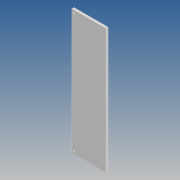
# Autodesk Inventor part: KB33-046-004-005 - Лицевая наклонная пластина
Saved by Autodesk Inventor 2020 (Build 240168000, 168)
## iProperties
Created: 2021-06-25
Part Number: KB33-046-004-005 - Лицевая наклонная пластина
Material: Типовые
Document SubType Name: Modeling
Designer: Петров Иван
Mass: 52.5036 g
Surface Area: 285.592 cm^2
Volume: 52.5036 cm^3
Density: 1 g/cm^3
Appearance: По умолчанию
Author: Петров Иван
Autodesk Inventor part; units mm, degrees
ref_plane "YZ Plane" through (0, 0, 0) normal (1, 0, 0) x (0, 1, 0)
ref_plane "XZ Plane" through (0, 0, 0) normal (0, 1, 0) x (-1, 0, 0)
ref_plane "XY Plane" through (0, 0, 0) normal (0, 0, 1) x (1, 0, 0)
sketch "Эскиз1" plane through (0, 0, 0) normal (0, 0, 1) x (1, 0, 0)
  circle A0 centre (3.6373, -187.3954) radius 1.5 projected
  circle A1 centre (3.6373, 22.3954) radius 1.5 projected
  line L0 (0, 27) -> (60, 27)
  line L1 (60, 27) -> (60, -190.5454)
  line L2 (60, -190.5454) -> (0, -190.5454)
  line L3 (0, -190.5454) -> (0, 27)
  point P0 (0, 0)
  point P1 (0, -190.5454)
  dimension "d0" = 60
  constraints: 8 end point, 2 parallel, 1 horizontal, 1 perpendicular, 2 other
  measures "d0" distance of L1.end L2.end
extrude "Выдавливание1" add sketch "Эскиз1" along normal blind 4
thicken "Толщина1" operation add thickness 1.455 both sides no extend neighbours yes toward (0, -1, 0) faces at (20, -190.5454, 2.6667)
